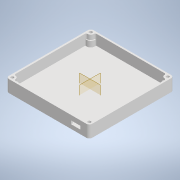
# Autodesk Inventor part: base
Saved by Autodesk Inventor 2021 (Build 250183000, 183)
## iProperties
Created: 2020-10-02
Part Number: base
Material: Generic
Document SubType Name: Modeling
Designer: ian66
Density: 1 g/cm^3
Appearance: Default
Author: ian66
Autodesk Inventor part; units mm, degrees
ref_plane "YZ Plane" through (0, 0, 0) normal (1, 0, 0) x (0, 1, 0)
ref_plane "XZ Plane" through (0, 0, 0) normal (0, 1, 0) x (-1, 0, 0)
ref_plane "XY Plane" through (0, 0, 0) normal (0, 0, 1) x (1, 0, 0)
sketch "bottom" plane through (0, 0, 0) normal (0, 1, 0) x (-1, 0, 0)
  line L0 (4.0046, -0.4434) -> (-83.9954, -0.4434)
  line L1 (-83.9954, -0.4434) -> (-83.9954, -89.9434)
  line L2 (-83.9954, -89.9434) -> (4.0046, -89.9434)
  line L3 (4.0046, -89.9434) -> (4.0046, -0.4434)
  line L4 (2.2046, -2.2434) -> (-82.1954, -2.2434)
  line L5 (-82.1954, -2.2434) -> (-82.1954, -88.1434)
  line L6 (-82.1954, -88.1434) -> (2.2046, -88.1434)
  line L7 (2.2046, -88.1434) -> (2.2046, -2.2434)
  circle A0 centre (0.4546, -3.9934) radius 3.55
  line L8 (-39.9954, -123.8489) -> (-39.9954, 33.4211)
  line L9 (23.3841, -45.1934) -> (-117.3219, -45.1934)
  circle A1 centre (0.4546, -3.9934) radius 1.75
  circle A2 centre (-80.4454, -3.9934) radius 3.55
  circle A3 centre (-80.4454, -3.9934) radius 1.75
  circle A4 centre (0.4546, -86.3934) radius 1.75
  circle A5 centre (0.4546, -86.3934) radius 3.55
  circle A6 centre (-80.4454, -86.3934) radius 1.75
  circle A7 centre (-80.4454, -86.3934) radius 3.55
  line L10 (3.6301, -3.9991) -> (2.0374, -6.7462)
  line L11 (2.0374, -6.7462) -> (-1.138, -6.7405)
  line L12 (-1.138, -6.7405) -> (-2.7208, -3.9877)
  line L13 (-2.7208, -3.9877) -> (-1.1282, -1.2406)
  line L14 (-1.1282, -1.2406) -> (2.0472, -1.2462)
  line L15 (2.0472, -1.2462) -> (3.6301, -3.9991)
  circle A8 centre (0.4546, -3.9934) radius 4.55
  point P0 (0, 0)
  point P1 (-39.9954, -45.1934)
  point P2 (-2.6341, -2.2434)
  point P3 (2.2046, -7.0821)
  point P4 (2.2046, -83.3047)
  point P5 (-2.6341, -88.1434)
  point P6 (-77.3567, -88.1434)
  point P7 (-82.1954, -83.3047)
  point P8 (-82.1954, -7.0821)
  point P9 (-77.3567, -2.2434)
  point P10 (-39.9954, -0.4434)
  point P11 (-39.9954, -2.2434)
  point P12 (2.2046, -45.1934)
  point P13 (4.0046, -45.1934)
  point P14 (-39.9954, -45.1934)
  point P15 (-3.7454, -2.2434)
  point P16 (2.2046, -8.1934)
  dimension "d0" = 88
  dimension "d1" = 89.5
  dimension "d2" = 84.4
  dimension "d3" = 85.9
  dimension "d4" = 1.8
  dimension "d5" = 1.8
  dimension "d6" = 7.1
  dimension "d7" = 3.55
  dimension "d8" = 3.55
  dimension "d9" = 3.5
  dimension "d10" = 88
  dimension "d11" = 89.5
  dimension "d12" = 44.75
  dimension "d13" = 44
  dimension "d33" = 2.75
  dimension "d36" = 9.1
  constraints: 32 end point, 9 centre point, 6 coincident, 6 symmetric about line, 4 parallel, 3 horizontal, 2 perpendicular, 1 vertical, 19 other
  measures "d0" distance of L2.end L1.end
  measures "d1" distance of L1.end L0.end
  measures "d2" distance of L6.end L5.end
  measures "d3" distance of L5.end L4.end
  measures "d4" distance between parallel lines of L3 L7
  measures "d5" distance between parallel lines of L2 L6
  measures "d6" diameter of A0
  measures "d7" distance from line of L3 A0.centre
  measures "d8" distance from line of L0 A0.centre
  measures "d9" diameter of A1
  measures "d10" diameter of L3 L8
  measures "d11" diameter of L2 L9
  measures "d12" distance from line of L2 point (-39.995, -45.193)
  measures "d13" distance from line of L1 point (-39.995, -45.193)
  measures "d33" distance from line of L15 point (0.455, -3.993)
  measures "d36" diameter of A8
ref_plane "Work Plane3" through (39.9954, 0, -45.1934) normal (0, 0, 1) x (1, 0, 0)
ref_plane "Work Plane4" through (39.9954, 0, -45.1934) normal (1, 0, 0) x (0, 1, 0)
extrude "Extrusion4" add sketch "bottom" along normal blind 12.8 contours L3 A8 L0 | A8 L3 A0 L0 | A0 L4 A8 L0 | A0 L7 L10 L15 L14 L13 L4 | A8 L4 L8 L0 | L3 A8 L7 A0 | L4 L13 L12 L11 L10 L7 A0 | L3 L9 L7 A8 | L13 L14 L15 L10 L7 L4 | L4 A1 L7 L10 L11 L12 L13 | L4 L7 A1
extrude "Extrusion5" add sketch "bottom" along normal blind 1.8 contours A0 L7 A8 L4 | A8 L7 L9 L8 L4
fillet "Fillet3" radius 3 1 edges at (-4.0046, 6.4, -0.4434)
fillet "Fillet4" radius 1.5 2 edges at (-2.2046, 7.3, -7.0821) (2.6341, 7.3, -2.2434)
extrude "Extrusion6" cut sketch "bottom" along normal blind 2.5 contours L13 L14 L15 L10 L7 L4 | L4 A1 L7 L10 L11 L12 L13 | L4 L7 A1
extrude "pcb hight" add sketch "bottom" along normal blind 7.8 contours A0 L7 A8 L4
mirror "Mirror3" about plane through (39.9954, 0, -45.1934) normal (0, 0, 1)
mirror "Mirror4" about plane through (39.9954, 0, -45.1934) normal (1, 0, 0)
sketch "Sketch4" plane through (-1.0046, 0, -0.4434) normal (0, 0, 1) x (1, 0, 0)
  line L0 (65.6777, 7.8088) -> (75.6777, 7.8088)
  line L1 (75.6777, 7.8088) -> (75.6777, 4.3088)
  line L2 (75.6777, 4.3088) -> (65.6777, 4.3088)
  line L3 (65.6777, 4.3088) -> (65.6777, 7.8088)
  point P0 (1.0046, 0)
  dimension "d39" = 10
  dimension "d40" = 3.5
  constraints: 8 end point, 2 parallel, 1 horizontal, 1 perpendicular
  measures "d39" distance of L1.end L2.end
  measures "d40" distance of L0.end L1.end
extrude "Extrusion8" cut sketch "Sketch4" against normal blind 1.8
equation "\"d2\" = d0 - 2 * d4"
equation "\"d3\" = d1 - 2 * d5"
equation "\"d5\" = d4"
equation "\"d6\" = 2 * d4 + d9"
equation "\"d7\" = 0.5 * d6"
equation "\"d8\" = 0.5 * d6"
equation "\"d10\" = d0"
equation "\"d11\" = d1"
equation "\"d12\" = 0.5 * d1"
equation "\"d13\" = 0.5 * d0"
equation "\"d29\" = d4"
body "Solid2"
